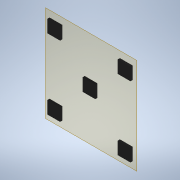
# Autodesk Inventor part: Part2
Saved by Autodesk Inventor 2020 (Build 240168000, 168)
## iProperties
Created: 2022-04-27
Part Number: Part2
Material: Generic
Document SubType Name: Modeling
Designer: Manish
Density: 1 g/cm^3
Appearance: Default
Author: Manish
Autodesk Inventor part; units mm, degrees
ref_plane "YZ Plane" through (0, 0, 0) normal (1, 0, 0) x (0, 1, 0)
ref_plane "XZ Plane" through (0, 0, 0) normal (0, 1, 0) x (-1, 0, 0)
ref_plane "XY Plane" through (0, 0, 0) normal (0, 0, 1) x (1, 0, 0)
ref_plane "Work Plane1" through (0, 0, 0) normal (0, 0, 1) x (1, 0, 0)
sketch "Sketch1" plane through (0, 0, 0) normal (0, 0, 1) x (1, 0, 0)
  line L0 (500, 500) -> (347.6, 500)
  line L1 (347.6, 500) -> (347.6, 347.6)
  line L2 (347.6, 347.6) -> (500, 347.6)
  line L3 (500, 347.6) -> (500, 500)
  line L4 (500, 500) -> (-500, 500)
  line L5 (-500, 500) -> (-500, -500)
  line L6 (-500, -500) -> (500, -500)
  line L7 (500, -500) -> (500, 500)
  line L8 (-500, 500) -> (-500, 347.6)
  line L9 (-500, 347.6) -> (-347.6, 347.6)
  line L10 (-347.6, 347.6) -> (-347.6, 500)
  line L11 (-347.6, 500) -> (-500, 500)
  line L12 (347.6, -347.6) -> (347.6, -500)
  line L13 (347.6, -500) -> (500, -500)
  line L14 (500, -500) -> (500, -347.6)
  line L15 (500, -347.6) -> (347.6, -347.6)
  line L16 (-500, -347.6) -> (-500, -500)
  line L17 (-500, -500) -> (-347.6, -500)
  line L18 (-347.6, -500) -> (-347.6, -347.6)
  line L19 (-347.6, -347.6) -> (-500, -347.6)
  line L20 (76.2, 101.6) -> (-76.2, 101.6)
  line L21 (-76.2, 101.6) -> (-76.2, -50.8)
  line L22 (-76.2, -50.8) -> (76.2, -50.8)
  line L23 (76.2, -50.8) -> (76.2, 101.6)
  point P0 (0, 0)
  dimension "d0" = 152.4
  dimension "d1" = 152.4
  dimension "d2" = 1000
  dimension "d3" = 1000
  dimension "d6" = 847.6
  dimension "d9" = 847.6
  dimension "d12" = 152.4
  dimension "d13" = 152.4
  constraints: 48 end point, 6 parallel, 4 horizontal, 3 perpendicular, 1 vertical, 24 other
  measures "d0" distance of L2.end L1.end
  measures "d1" distance of L1.end L0.end
  measures "d2" distance of L6.end L5.end
  measures "d3" distance of L5.end L4.end
  measures "d6" distance of L0.end L8.start
  measures "d9" distance of L0.end L12.start
  measures "d12" distance of L22.end L21.end
  measures "d13" distance of L21.end L20.end
extrude "Extrusion1" add sketch "Sketch1" along normal blind 25.4 contours L3 L2 L1 L0 | L10 L9 L5 L4 | L7 L6 L12 L15 | L19 L18 L6 L5 | L23 L22 L21 L20
body "Solid1"
